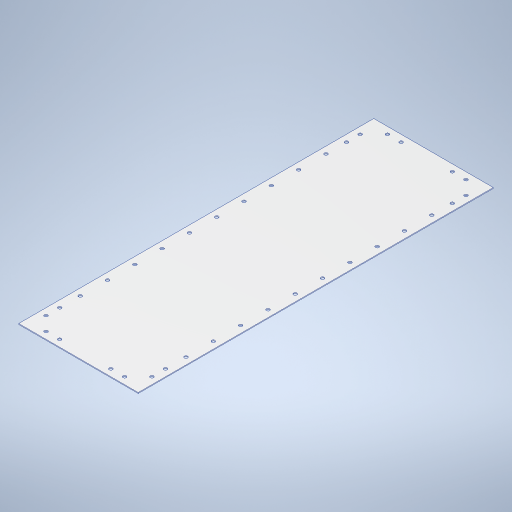
# Autodesk Inventor part: Centerpiece_bottomPlate
Saved by Autodesk Inventor 2023 (Build 270158000, 158)
## iProperties
Created: 2022-10-10
Part Number: Centerpiece_bottomPlate
Material: Aluminum 6061
Document SubType Name: Modeling
Designer: Nebil
Density: 2.7 g/cm^3
Appearance: Aluminum - Flat
Author: Nebil
Autodesk Inventor part; units mm, degrees
ref_plane "YZ Plane" through (0, 0, 0) normal (1, 0, 0) x (0, 1, 0)
ref_plane "XZ Plane" through (0, 0, 0) normal (0, 1, 0) x (-1, 0, 0)
ref_plane "XY Plane" through (0, 0, 0) normal (0, 0, 1) x (1, 0, 0)
sketch "Sketch1" plane through (0, 0, 0) normal (0, 1, 0) x (-1, 0, 0)
  line L0 (-111.125, -330.2) -> (111.125, -330.2)
  line L1 (111.125, -330.2) -> (111.125, 330.2)
  line L2 (111.125, 330.2) -> (-111.125, 330.2)
  line L3 (-111.125, 330.2) -> (-111.125, -330.2)
  line L4 (-111.125, -330.2) -> (111.125, 330.2) construction
  line L5 (111.125, -330.2) -> (-111.125, 330.2) construction
  point P0 (0, 0)
  dimension "d0" = 222.25
  dimension "d1" = 660.4
  constraints: 12 end point, 2 midpoint, 2 parallel, 1 horizontal, 1 perpendicular
  measures "d0" distance of L2.end L1.end
  measures "d1" distance of L1.end L0.end
extrude "Extrusion1" add sketch "Sketch1" along normal blind 1.5875
sketch "Sketch2" plane through (0, 1.5875, 0) normal (0, 1, 0) x (1, 0, 0)
  line L0 (-111.125, 330.2) -> (-111.125, -330.2) construction
  line L1 (-111.125, -304.8) -> (111.125, -304.8) construction
  line L2 (111.125, -330.2) -> (111.125, 330.2) construction
  line L3 (-111.125, -330.2) -> (111.125, -330.2) construction
  line L4 (-111.125, 304.8) -> (111.125, 304.8) construction
  line L5 (111.125, 330.2) -> (-111.125, 330.2) construction
  line L6 (85.725, 330.2) -> (85.725, -344.7266) construction
  line L7 (-85.725, 330.2) -> (-85.725, -330.2) construction
  circle A0 centre (98.425, -292.1) radius 3.175
  line L8 (-111.125, 0) -> (111.125, 0) construction
  circle A1 centre (73.025, -317.5) radius 3.175
  line L9 (0, 330.2) -> (0, -330.2) construction
  point P0 (0, 0)
  dimension "d4" = 25.4
  dimension "d5" = 25.4
  dimension "d6" = 25.4
  dimension "d7" = 25.4
  dimension "d8" = 6.35
  dimension "d9" = 12.7
  dimension "d10" = 12.7
  dimension "d11" = 6.35
  dimension "d12" = 12.7
  dimension "d13" = 12.7
  constraints: 12 end point, 7 point on line, 4 midpoint, 3 perpendicular, 2 centre point, 1 horizontal
  measures "d4" distance between parallel lines of L3 L1
  measures "d5" distance between parallel lines of L4 L5
  measures "d6" distance between parallel lines of L2 L6
  measures "d7" distance between parallel lines of L0 L7
  measures "d8" diameter of A0
  measures "d9" distance from line of A0.centre L6
  measures "d10" distance from line of L1 A0.centre
  measures "d11" diameter of A1
  measures "d12" distance from line of A1.centre L1
  measures "d13" distance from line of L6 A1.centre
extrude "Extrusion2" cut sketch "Sketch2" against normal through all contours A1
extrude "Extrusion3" cut sketch "Sketch2" against normal blind 25.4 contours A0
pattern_linear "Rectangular Pattern3" count 2 spacing 25.4 along (-1, 0, 0) of "Extrusion2"
pattern_linear "Rectangular Pattern2" count 2 spacing 25.4 along (0, 0, -1) of "Extrusion3"
mirror "Mirror2" about plane through (0, 0, 0) normal (1, 0, 0) of "Extrusion3", "Rectangular Pattern2", "Extrusion2", "Rectangular Pattern3"
sketch "Sketch3" plane through (0, 1.5875, 0) normal (0, 1, 0) x (1, 0, 0)
  circle A0 centre (98.425, -266.7) radius 3.175 projected
  circle A1 centre (98.425, -228.6) radius 3.175
  line L0 (111.125, -330.2) -> (111.125, 330.2) projected
  circle A2 centre (98.425, -177.8) radius 3.175
  circle A3 centre (98.425, -127) radius 3.175
  circle A4 centre (98.425, -76.2) radius 3.175
  circle A5 centre (98.425, -25.4) radius 3.175
  circle A6 centre (98.425, 25.4) radius 3.175
  circle A7 centre (98.425, 76.2) radius 3.175
  circle A8 centre (98.425, 127) radius 3.175
  circle A9 centre (98.425, 177.8) radius 3.175
  circle A10 centre (98.425, 228.6) radius 3.175
  point P0 (0, 0)
  dimension "d24" = 6.35
  dimension "d25" = 6.35
  dimension "d26" = 38.1
  dimension "d29" = 50.8
  constraints: 10 centre point, 1 vertical, 1 vertical alignment, 18 other
  measures "d24" diameter of A0
  measures "d25" diameter of A1
  measures "d26" distance of A0.centre A1.centre
  measures "d29" distance of A1.centre A2.centre
extrude "Extrusion4" cut sketch "Sketch3" against normal blind 25.4 contours A1 | A2 | A3 | A4 | A5 | A6 | A7 | A8 | A9 | A10
mirror "Mirror3" about plane through (0, 0, 0) normal (1, 0, 0) of "Extrusion4"
mirror "Mirror4" about plane through (0, 0, 0) normal (0, 0, 1) of "Rectangular Pattern3", "Rectangular Pattern2", "Extrusion3", "Extrusion2", "Mirror2"
equation "\"d25\" = d24"
body "Solid1"
